Autodesk Fusion 360 part; units mm, degrees
(part 2 of 2)
sketch "Sketch1 (6)" plane through (0, 0, 0) normal (0, 1, 0) x (1, 0, 0) in component "Peça P3"
  line L0 (-20, -6) -> (-20, 10)
  line L1 (36, 30) -> (-36, 30)
  line L2 (-20, 10) -> (20, 10)
  line L3 (40, -6) -> (40, 26)
  arc A0 (-40, -6) -> (-36, -10) centre (-36, -6) ccw
  arc A1 (20, -6) -> (24, -10) centre (24, -6) ccw
  arc A2 (-24, -10) -> (-20, -6) centre (-24, -6) ccw
  line L4 (-40, 26) -> (-40, -6)
  line L5 (20, 10) -> (20, -6)
  arc A3 (-36, 30) -> (-40, 26) centre (-36, 26) ccw
  arc A4 (40, 26) -> (36, 30) centre (36, 26) ccw
  line L6 (24, -10) -> (36, -10)
  arc A5 (36, -10) -> (40, -6) centre (36, -6) ccw
  line L7 (-36, -10) -> (-24, -10)
  point P0 (-20, -10)
  point P1 (40, -10)
  point P2 (-40, -10)
  point P3 (-40, 30)
  dimension "d21" = 80
  dimension "d22" = 40
  dimension "d23" = 40
  dimension "d24" = 20
  dimension "d25" = 4
  dimension "d26" = 4
  dimension "d27" = 4
  dimension "d28" = 4
  dimension "d29" = 4
  dimension "d30" = 4
  constraint horizontal L1
  constraint perpendicular L1 L4
  constraint parallel L1 L7
  constraint parallel L3 L4
  constraint parallel L0 L5
  constraint coincident P3 L1
  constraint coincident P3 L4
  constraint tangent L1 A3
  constraint tangent L4 A3
  constraint tangent L1 A4
  constraint tangent L3 A4
  constraint collinear L6 L7
  constraint coincident P0 L0
  constraint coincident P0 L7
  constraint tangent L0 A2
  constraint tangent A2 L7
  constraint tangent A1 L5
  constraint tangent A1 L6
  constraint coincident P1 L3
  constraint coincident P1 L6
  constraint tangent L3 A5
  constraint tangent L6 A5
  constraint coincident P2 L4
  constraint coincident P2 L7
  constraint tangent A0 L4
  constraint tangent A0 L7
  measures "d21" distance of P1 P2
  measures "d22" distance of P2 P3
  measures "d23" distance of L2.end L0.end
  measures "d24" distance of P0 L0.end
  measures "d25" radius of A3
  measures "d26" radius of A4
  measures "d27" radius of A2
  measures "d28" radius of A1
  measures "d29" radius of A5
  measures "d30" radius of A0
extrude "Extrude2" add sketch "Sketch1" along normal blind 15 makes body 1 in component "Peça P1"
extrude "Extrude2'" add sketch "Sketch1 (2)" along normal blind 15 separate body makes body 2 in component "Peça P2"
extrude "Extrude2''" add sketch "Sketch1 (3)" along normal blind 15 separate body makes body 3 in component "Peça P3"
extrude "Extrude2'''" add sketch "Sketch1 (4)" along normal blind 15 separate body makes body 4 in component "Peça P4"
extrude "Extrude2''''" add sketch "Sketch1 (5)" along normal blind 15 separate body makes body 5 in component "Peça G1"
extrude "Extrude1" add sketch "Sketch G2" along normal blind 15 separate body makes body 6 in component "Peça G2"
extrude "Extrude1'" add sketch "Sketch G3" along normal blind 15 separate body makes body 7 in component "Peça G3"
extrude "Extrude1''" add sketch "Sketch G4" along normal blind 15 separate body makes body 8 in component "Peça G4"
sketch "Sketch C1" plane through (0, 0, 0) normal (0, 1, 0) x (1, 0, 0) in component "Peça C1"
  line L0 (-40.0297, 4.2229) -> (-40.0318, 36.0014)
  line L1 (-36.0335, 40.0017) -> (-4.255, 40.0151)
  arc A0 (-0.2817, 44.4612) -> (-44.4739, 0.2474) centre (-40.0321, 40) ccw
  arc A1 (-4.255, 40.0151) -> (-0.2817, 44.4612) centre (-4.2567, 44.0151) ccw
  arc A2 (-36.0335, 40.0017) -> (-40.0318, 36.0014) centre (-36.0318, 36.0017) ccw
  arc A3 (-44.4739, 0.2474) -> (-40.0297, 4.2229) centre (-44.0297, 4.2226) ccw
  line L2 (-65, 60) -> (-65, 25)
  line L3 (-70, 25) -> (-70, 60)
  line L4 (-45, 70) -> (-45, 45)
  line L5 (-50, 45) -> (-50, 70)
  line L6 (-30, 75) -> (-30, 45)
  line L7 (-35, 45) -> (-35, 75)
  line L8 (-55, 65) -> (-55, 35)
  line L9 (-60, 35) -> (-60, 65)
  arc A4 (-30, 75) -> (-35, 75) centre (-32.5, 75) ccw
  arc A5 (-35, 45) -> (-30, 45) centre (-32.5, 45) ccw
  arc A6 (-50, 45) -> (-45, 45) centre (-47.5, 45) ccw
  arc A7 (-45, 70) -> (-50, 70) centre (-47.5, 70) ccw
  arc A8 (-55, 65) -> (-60, 65) centre (-57.5, 65) ccw
  arc A9 (-60, 35) -> (-55, 35) centre (-57.5, 35) ccw
  arc A10 (-70, 25) -> (-65, 25) centre (-67.5, 25) ccw
  arc A11 (-65, 60) -> (-70, 60) centre (-67.5, 60) ccw
  point P0 (-40.0294, 0)
  point P1 (-40.0321, 40)
  point P2 (0, 20)
  dimension "d415" = 40
  dimension "d416" = 4
  dimension "d417" = 4
  dimension "d418" = 4
  dimension "d419" = 2.5
  dimension "d420" = 4.2567
  dimension "d421" = 15.9849
  dimension "d422" = 9.0151
  dimension "d423" = 0.9849
  dimension "d424" = 63.2433
  dimension "d425" = 53.2433
  dimension "d426" = 43.2433
  dimension "d427" = 28.2433
  dimension "d428" = 89.976
  dimension "d429" = 30
  dimension "d430" = 25
  dimension "d431" = 24.0151
  dimension "d432" = 39.7924
  dimension "d433" = 35
  constraint coincident P1 A0.centre
  constraint tangent A0 A1
  constraint tangent L1 A1
  constraint coincident P1 L0
  constraint coincident P1 L1
  constraint tangent L0 A2
  constraint tangent L1 A2
  constraint coincident P0 L0
  constraint coincident P0 A0
  constraint tangent L0 A3
  constraint tangent A0 A3
  constraint vertical L2
  constraint vertical L3
  constraint vertical L4
  constraint vertical L5
  constraint vertical L6
  constraint vertical L7
  constraint vertical L8
  constraint vertical L9
  constraint tangent L3 A11
  constraint tangent L3 A10
  constraint tangent L9 A8
  constraint tangent L9 A9
  constraint tangent L4 A7
  constraint tangent L5 A6
  constraint tangent L7 A4
  constraint tangent L6 A5
  constraint tangent L2 A10
  constraint tangent L2 A11
  constraint tangent L8 A9
  constraint tangent L8 A8
  constraint tangent L5 A7
  constraint tangent L4 A6
  constraint tangent L7 A5
  constraint tangent L6 A4
  constraint horizontal L5.start L7.start
  constraint equal A4 A6
  constraint equal A4 A8
  constraint equal A4 A10
  constraint equal L6 L8
  constraint vertical origin P2
  constraint horizontal origin P0
  measures "d415" distance of P0 A0.centre
  measures "d416" radius of A1
  measures "d417" radius of A2
  measures "d418" radius of A3
  measures "d419" radius of A5
  measures "d420" horizontal distance of origin A1.centre
  measures "d421" vertical distance of A1.centre A11.centre
  measures "d422" vertical distance of A1.centre A9.centre
  measures "d423" vertical distance of A1.centre A5.centre
  measures "d424" horizontal distance of A1.centre A11.centre
  measures "d425" horizontal distance of A1.centre A9.centre
  measures "d426" horizontal distance of A1.centre A6.centre
  measures "d427" horizontal distance of A1.centre A5.centre
  measures "d428" angle of L1 L3
  measures "d429" vertical distance of A4.centre A5.centre
  measures "d430" vertical distance of A7.centre A6.centre
  measures "d431" vertical distance of P2 A1.centre
  measures "d432" vertical distance of A1.centre A3.centre
  measures "d433" vertical distance of A11.centre A10.centre
sketch "Sketch C2" plane through (0, 0, 0) normal (0, 1, 0) x (1, 0, 0) in component "Peça C2"
  arc A0 (-44.4661, 0.2446) -> (-40.0232, 4.2216) centre (-44.0232, 4.22) ccw
  line L0 (-40.0232, 4.2216) -> (-40.0355, 35.9987)
  line L1 (-36.037, 40.0002) -> (-4.2599, 40.0124)
  arc A1 (-4.2599, 40.0124) -> (-0.2864, 44.4584) centre (-4.2615, 44.0124) ccw
  arc A2 (-0.2864, 44.4584) -> (-44.4661, 0.2446) centre (-40.037, 39.9987) ccw
  arc A3 (-36.037, 40.0002) -> (-40.0355, 35.9987) centre (-36.0355, 36.0002) ccw
  circle A4 centre (-59.1399, 63.4514) radius 5
  circle A5 centre (-45.0248, 68.2909) radius 5
  circle A6 centre (-66.8025, 53.3691) radius 3
  circle A7 centre (-47.0412, 53.7724) radius 3
  circle A8 centre (-49.0577, 13.0401) radius 5
  circle A9 centre (-61.7613, 37.2375) radius 5
  circle A10 centre (-33.7327, 60.6284) radius 3
  circle A11 centre (-13.1649, 50.3445) radius 6
  circle A12 centre (-52.8889, 45.9083) radius 4
  circle A13 centre (-27.0784, 67.2827) radius 4
  circle A14 centre (-29.2965, 49.9412) radius 4
  circle A15 centre (-73.0535, 43.8918) radius 3
  circle A16 centre (-49.8643, 28.5668) radius 5
  circle A17 centre (-64.3827, 23.929) radius 4
  circle A18 centre (-71.4403, 32.5997) radius 4
  point P0 (-40.037, 39.9987)
  point P1 (-40.0216, -0.0013)
  point P2 (-0.0047, 19.9974)
  point P3 (-0.0047, -0.0013)
  dimension "d434" = 40
  dimension "d435" = 4
  dimension "d436" = 4
  dimension "d437" = 4
  dimension "d439" = 4.2567
  dimension "d450" = 24.0151
  dimension "d451" = 39.7924
  dimension "d453" = 10
  dimension "d454" = 10
  dimension "d455" = 6
  dimension "d456" = 6
  dimension "d457" = 10
  dimension "d458" = 10
  dimension "d459" = 6
  dimension "d460" = 12
  dimension "d461" = 8
  dimension "d462" = 8
  dimension "d463" = 8
  dimension "d464" = 6
  dimension "d465" = 10
  dimension "d466" = 8
  dimension "d467" = 8
  dimension "d468" = 4.2615
  dimension "d469" = 67.1788
  dimension "d470" = 62.541
  dimension "d471" = 60.1213
  dimension "d472" = 57.4999
  dimension "d473" = 54.8785
  dimension "d474" = 48.6275
  dimension "d475" = 45.6028
  dimension "d476" = 44.7962
  dimension "d477" = 42.7798
  dimension "d478" = 40.7633
  dimension "d479" = 29.4712
  dimension "d480" = 25.035
  dimension "d481" = 22.8169
  dimension "d482" = 8.9034
  dimension "d483" = 90
  dimension "d484" = 44.0124
  dimension "d485" = 68.792
  dimension "d486" = 30.9723
  dimension "d487" = 24.2784
  dimension "d488" = 23.2702
  dimension "d489" = 20.0835
  dimension "d490" = 19.439
  dimension "d491" = 16.6159
  dimension "d492" = 15.4457
  dimension "d493" = 11.4128
  dimension "d494" = 9.76
  dimension "d495" = 9.3567
  dimension "d496" = 6.7749
  dimension "d497" = 6.332
  dimension "d498" = 5.9287
  dimension "d499" = 1.8958
  dimension "d500" = 0.1206
  constraint coincident P0 A2.centre
  constraint tangent A1 A2
  constraint tangent L1 A1
  constraint coincident P0 L0
  constraint coincident P0 L1
  constraint tangent L0 A3
  constraint tangent L1 A3
  constraint coincident P1 L0
  constraint coincident P1 A2
  constraint tangent A0 L0
  constraint tangent A0 A2
  constraint vertical P2 P3
  constraint horizontal P1 P3
  measures "d434" distance of P0 P1
  measures "d435" radius of A1
  measures "d436" radius of A3
  measures "d437" radius of A0
  measures "d439" horizontal distance of A1.centre P3
  measures "d450" vertical distance of P2 A1.centre
  measures "d451" vertical distance of A1.centre A0.centre
  measures "d453" diameter of A4
  measures "d454" diameter of A5
  measures "d455" diameter of A6
  measures "d456" diameter of A7
  measures "d457" diameter of A8
  measures "d458" diameter of A9
  measures "d459" diameter of A10
  measures "d460" diameter of A11
  measures "d461" diameter of A12
  measures "d462" diameter of A13
  measures "d463" diameter of A14
  measures "d464" diameter of A15
  measures "d465" diameter of A16
  measures "d466" diameter of A17
  measures "d467" diameter of A18
  measures "d468" horizontal distance of origin A1.centre
  measures "d469" horizontal distance of A1.centre A18.centre
  measures "d470" horizontal distance of A1.centre A6.centre
  measures "d471" horizontal distance of A1.centre A17.centre
  measures "d472" horizontal distance of A1.centre A9.centre
  measures "d473" horizontal distance of A1.centre A4.centre
  measures "d474" horizontal distance of A1.centre A12.centre
  measures "d475" horizontal distance of A1.centre A16.centre
  measures "d476" horizontal distance of A1.centre A8.centre
  measures "d477" horizontal distance of A1.centre A7.centre
  measures "d478" horizontal distance of A1.centre A5.centre
  measures "d479" horizontal distance of A1.centre A10.centre
  measures "d480" horizontal distance of A1.centre A14.centre
  measures "d481" horizontal distance of A1.centre A13.centre
  measures "d482" horizontal distance of A1.centre A11.centre
  measures "d483" angle of L0 L1
  measures "d484" vertical distance of origin A1.centre
  measures "d485" horizontal distance of A1.centre A15.centre
  measures "d486" vertical distance of A1.centre A8.centre
  measures "d487" vertical distance of A1.centre A5.centre
  measures "d488" vertical distance of A1.centre A13.centre
  measures "d489" vertical distance of A1.centre A17.centre
  measures "d490" vertical distance of A1.centre A4.centre
  measures "d491" vertical distance of A1.centre A10.centre
  measures "d492" vertical distance of A1.centre A16.centre
  measures "d493" vertical distance of A1.centre A18.centre
  measures "d494" vertical distance of A1.centre A7.centre
  measures "d495" vertical distance of A1.centre A6.centre
  measures "d496" vertical distance of A1.centre A9.centre
  measures "d497" vertical distance of A1.centre A11.centre
  measures "d498" vertical distance of A1.centre A14.centre
  measures "d499" vertical distance of A1.centre A12.centre
  measures "d500" vertical distance of A1.centre A15.centre
sketch "Sketch C3" plane through (0, 0, 0) normal (0, 1, 0) x (1, 0, 0) in component "Peça C3"
  arc A0 (-4.2599, 40.0124) -> (-0.2864, 44.4584) centre (-4.2615, 44.0124) ccw
  arc A1 (-0.2864, 44.4584) -> (-44.4661, 0.2446) centre (-40.037, 39.9987) ccw
  line L0 (-36.037, 40.0002) -> (-4.2599, 40.0124)
  arc A2 (-36.037, 40.0002) -> (-40.0355, 35.9987) centre (-36.0355, 36.0002) ccw
  arc A3 (-44.4661, 0.2446) -> (-40.0232, 4.2216) centre (-44.0232, 4.22) ccw
  line L1 (-40.0232, 4.2216) -> (-40.0355, 35.9987)
  arc A4 (-4.8251, 44.5122) -> (-44.5234, 4.7833) centre (-40.037, 39.9987) ccw
  line L2 (-44.5234, 4.7833) -> (-44.5355, 35.9969)
  arc A5 (-36.0387, 44.5002) -> (-44.5355, 35.9969) centre (-36.0355, 36.0002) ccw
  line L3 (-36.0387, 44.5002) -> (-4.8251, 44.5122)
  point P0 (-40.0216, -0.0013)
  point P1 (-0.0047, 19.9974)
  point P2 (-40.037, 39.9987)
  point P3 (-0.0047, -0.0013)
  dimension "d501" = 40
  dimension "d502" = 4
  dimension "d503" = 4
  dimension "d504" = 4
  dimension "d505" = 4.2567
  dimension "d506" = 24.0151
  dimension "d507" = 39.7924
  dimension "d523" = 4.2615
  dimension "d538" = 90
  dimension "d539" = 44.0124
  dimension "d556" = -4.5
  constraint coincident P2 A1.centre
  constraint tangent A0 A1
  constraint tangent A0 L0
  constraint coincident P2 L1
  constraint coincident P2 L0
  constraint tangent A2 L1
  constraint tangent L0 A2
  constraint coincident P0 L1
  constraint coincident P0 A1
  constraint tangent A3 L1
  constraint tangent A1 A3
  constraint vertical P1 P3
  constraint horizontal P0 P3
  measures "d501" distance of P0 P2
  measures "d502" radius of A0
  measures "d503" radius of A2
  measures "d504" radius of A3
  measures "d505" horizontal distance of P3 A0.centre
  measures "d506" vertical distance of P1 A0.centre
  measures "d507" vertical distance of A3.centre A0.centre
  measures "d523" horizontal distance of origin A0.centre
  measures "d538" angle of L0 L1
  measures "d539" vertical distance of origin A0.centre
extrude "Extrude1'''" add sketch "Sketch C1" along normal blind 15 separate body makes body 9 in component "Peça C1"
extrude "Extrude1''''" add sketch "Sketch C2" along normal blind 15 separate body makes body 10 in component "Peça C2"
extrude "Extrude1'''''" add sketch "Sketch C3" along normal blind 15 separate body makes body 11 in component "Peça C3"
other "Arrange1"
move_body "Move1" bodies 3 to x (-1, 0, 0) y (0, 1, 0) z (0, 0, -1) at (-80, 0, -60) in component "Peça P3"
move_body "Move1'" bodies 4 to x (0, 0, -1) y (0, 1, 0) z (1, 0, 0) at (-10, 0, -70) in component "Peça P4"
move_body "Move2" bodies 4 to x (0, 0, -1) y (0, 1, 0) z (1, 0, 0) at (70, 0, -150) in component "Peça P4"
move_body "Move3" bodies 4 to x (1, 0, 0) y (0, 1, 0) z (0, 0, 1) at (0, 0, 250) in component "Peça P4"
move_body "Move1''" bodies 5 to x (-1, 0, 0) y (0, 1, 0) z (0, 0, -1) at (-221, 0, -80) in component "Peça G1"
move_body "Move2'" bodies 3 to x (0, 1, 0) y (-1, 0, 0) z (0, 0, 1) at (-140, 140, 0) in component "Peça P3"
move_body "Move1'''" bodies 2 to x (0, 1, 0) y (-1, 0, 0) z (0, 0, 1) at (-101.7071, 101.7071, 0) in component "Peça P2"
move_body "Move4" bodies 4 to x (0, 1, 0) y (-1, 0, 0) z (0, 0, 1) at (-101.7071, 101.7071, 0) in component "Peça P4"
move_body "Move2''" bodies 5 to x (0, 1, 0) y (-1, 0, 0) z (0, 0, 1) at (-230.5, 230.5, 0) in component "Peça G1"
move_body "Move2'''" bodies 2 to x (1, 0, 0) y (0, 1, 0) z (0, 0, 1) at (0, -2, 0) in component "Peça P2"
move_body "Move5" bodies 4 to x (1, 0, 0) y (0, 1, 0) z (0, 0, 1) at (0, -1, 0) in component "Peça P4"
move_body "Move3'" bodies 2 to x (1, 0, 0) y (0, 1, 0) z (0, 0, 1) at (0, 0.5, 0) in component "Peça P2"
move_body "Move6" bodies 4 to x (1, 0, 0) y (0, 1, 0) z (0, 0, 1) at (0, -0.5, 0) in component "Peça P4"
move_body "Move3''" bodies 3 to x (1, 0, 0) y (0, 1, 0) z (0, 0, 1) at (0, -60, -100) in component "Peça P3"
move_body "Move4'" bodies 2 to x (1, 0, 0) y (0, 1, 0) z (0, 0, 1) at (0, -60, -100) in component "Peça P2"
move_body "Move7" bodies 4 to x (1, 0, 0) y (0, 1, 0) z (0, 0, 1) at (0, 60, 100) in component "Peça P4"
move_body "Move3'''" bodies 5 to x (1, 0, 0) y (0, 1, 0) z (0, 0, 1) at (0, -60, -100) in component "Peça G1"
move_body "Move1''''" bodies 9 to x (1, 0, 0) y (0, 1, 0) z (0, 0, 1) at (150, 0, 0) in component "Peça C1"
move_body "Move2''''" bodies 9 to x (-1, 0, 0) y (0, 1, 0) z (0, 0, -1) at (139.9358, 0, 10) in component "Peça C1"
move_body "Move1'''''" bodies 6 to x (1, 0, 0) y (0, 1, 0) z (0, 0, 1) at (0, 0, 150) in component "Peça G2"
move_body "Move2'''''" bodies 6 to x (0, 0, 1) y (0, 1, 0) z (-1, 0, 0) at (-0.5, 0, 220.5) in component "Peça G2"
move_body "Move3''''" bodies 6 to x (1, 0, 0) y (0, 1, 0) z (0, 0, 1) at (40, 0, -50) in component "Peça G2"
move_body "Move4''" bodies 6 to x (1, 0, 0) y (0, 1, 0) z (0, 0, 1) at (0, 0, -10) in component "Peça G2"
move_body "Move1''''''" bodies 1 to x (1, 0, 0) y (0, 1, 0) z (0, 0, 1) at (0, 90, 0) in component "Peça P1"
move_body "Move2''''''" bodies 1 to x (1, 0, 0) y (0, 1, 0) z (0, 0, 1) at (-180, 0, 0) in component "Peça P1"
move_body "Move3'''''" bodies 1 to x (1, 0, 0) y (0, 0, -1) z (0, 1, 0) at (280, 120, 60) in component "Peça P1"
move_body "Move4'''" bodies 1 to x (1, 0, 0) y (0, 1, 0) z (0, 0, 1) at (10, 0, 0) in component "Peça P1"
move_body "Move1'''''''" bodies 7 to x (1, 0, 0) y (0, 0, 1) z (0, -1, 0) at (-50, -40, -40) in component "Peça G3"
move_body "Move2'''''''" bodies 7 to x (1, 0, 0) y (0, 1, 0) z (0, 0, 1) at (-1, 0, 0) in component "Peça G3"
move_body "Move1''''''''" bodies 8 to x (1, 0, 0) y (0, 1, 0) z (0, 0, 1) at (0, 0, 210) in component "Peça G4"
move_body "Move2''''''''" bodies 8 to x (0, 1, 0) y (-1, 0, 0) z (0, 0, 1) at (-110.5, 110.5, 0) in component "Peça G4"
move_body "Move3''''''" bodies 8 to x (-1, 0, 0) y (0, 1, 0) z (0, 0, -1) at (-251, 0, 340) in component "Peça G4"
move_body "Move4''''" bodies 8 to x (1, 0, 0) y (0, 1, 0) z (0, 0, 1) at (0, 0, 50) in component "Peça G4"
move_body "Move5'" bodies 8 to x (1, 0, 0) y (0, 1, 0) z (0, 0, 1) at (0, 0, -30) in component "Peça G4"
move_body "Move1'''''''''" bodies 10 to x (0, 0, 1) y (0, 1, 0) z (-1, 0, 0) at (-50.0357, 0, 0.0383) in component "Peça C2"
move_body "Move2'''''''''" bodies 10 to x (1, 0, 0) y (0, 1, 0) z (0, 0, 1) at (0, 0, 11.5) in component "Peça C2"
move_body "Move1''''''''''" bodies 11 to x (0, 1, 0) y (-1, 0, 0) z (0, 0, 1) at (-80.037, 80.037, 0) in component "Peça C3"
move_body "Move2''''''''''" bodies 11 to x (1, 0, 0) y (0, 0, 1) z (0, -1, 0) at (0, -79.9987, -79.9987) in component "Peça C3"
move_body "Move3'''''''" bodies 11 to x (1, 0, 0) y (0, 1, 0) z (0, 0, 1) at (0, 100, 150) in component "Peça C3"
move_body "Move3''''''''" bodies 10 to x (1, -0.000385, -0.000385) y (0.000385, 0, 1) z (-0.000385, -1, 0) at (0.0366, 125.0031, 95.0031) in component "Peça C2"
move_body "Move4'''''" bodies 11 to x (0, 0, -1) y (0, 1, 0) z (1, 0, 0) at (-165.0383, 0, -25.0357) in component "Peça C3"
move_body "Move4''''''" bodies 3 to x (0, 0, -1) y (0, 1, 0) z (1, 0, 0) at (-104.0059, 0, -205.9941) in component "Peça P3"
move_body "Move5''" bodies 1 to x (0, 0.000067, -1) y (-0.000067, 1, 0.000067) z (1, 0.000067, 0) at (140.0056, -0.0054, 79.9935) in component "Peça P1"
move_body "Move5'''" bodies 2 to x (0, 0, -1) y (0, 1, 0) z (1, 0, 0) at (-125.0059, 0, -108.4083) in component "Peça P2"
move_body "Move8" bodies 4 to x (0, 0, 1) y (0, 1, 0) z (-1, 0, 0) at (-15.0059, 0, 218.4083) in component "Peça P4"
move_body "Move6'" bodies 8 to x (0, 0, -1) y (0, 1, 0) z (1, 0, 0) at (-250.4996, 0, -30.5005) in component "Peça G4"
move_body "Move5''''" bodies 6 to x (1, 0, 0) y (0, 0, 1) z (0, -1, 0) at (0, 125.0069, 95.0069) in component "Peça G2"
move_body "Move3'''''''''" bodies 7 to x (0, -0.000067, -1) y (0.000067, 1, -0.000067) z (1, -0.000067, 0) at (-61.4956, -0.0095, -141.5035) in component "Peça G3"
move_body "Move3''''''''''" bodies 9 to x (1, 0, 0) y (0, 0, 1) z (0, -1, 0) at (0, 125.0069, 95.0069) in component "Peça C1"
move_body "Move4'''''''" bodies 5 to x (0, 0, -1) y (0, 1, 0) z (1, 0, 0) at (-165.5059, 0, -325.4941) in component "Peça G1"
extrude "Extrude1''''''" add 1 faces at (-95.5, -32.4931, 100.0069) faces seen with x (0, 1, 0.000067) y (-1, 0, 0) z (0, -0.000067, 1) at (-95.5, 110.5038, 0) along direction (1, 0, 0) blind 275 separate body on bodies 6 makes body 12 in component "Light for render"
move_body "Move1'''''''''''" bodies 12 to x (1, 0, 0) y (0, 1, 0) z (0, 0, 1) at (0, 175, 250) in component "Light for render"
extrude "Extrude2'''''" add 1 faces at (120.3264, 209.9971, 350.0019) along direction (0, 1, 0.000067) blind 275 on bodies 12 bodies 12 in component "Light for render"
move_body "Move2'''''''''''" bodies 12 to x (0.707107, 0, 0.707107) y (0, 1, 0) z (-0.707107, 0, 0.707107) at (-274.5025, 0, 145.6008) in component "Light for render"
move_body "Move3'''''''''''" bodies 12 to x (1, 0, 0) y (0, 1, 0) z (0, 0, 1) at (0, 0, 100) in component "Light for render"
move_body "Move4''''''''" bodies 12 to x (0.906308, -0.422618, 0) y (0.422618, 0.906308, 0) z (0, 0, 1) at (-129.8142, -225.5614, 0) in component "Light for render"
move_body "Move5'''''" bodies 12 to x (1, 0, 0) y (0, 0.906308, -0.422618) z (0, 0.422618, 0.906308) at (0, -29.3209, 81.1354) in component "Light for render"
move_body "Move6''" bodies 12 to x (1, 0, 0) y (0, 1, 0) z (0, 0, 1) at (0, 0, 300) in component "Light for render"
move_body "Move7'" bodies 12 to x (1, 0, 0) y (0, 1, 0) z (0, 0, 1) at (0, 0, 300) in component "Light for render"
move_body "Move8'" bodies 12 to x (-0.173648, 0, -0.984808) y (-0.336824, 0.939693, 0.059391) z (0.925417, 0.34202, -0.163176) at (-792.9971, -286.4144, 455.4732) in component "Light for render"
component "Peça P2" placed x (1, 0, 0) y (0, 1, 0.000067) z (0, -0.000067, 1) at (6.2071, 80.2041, 101.7061)
component "Peça P3" placed x (1, 0, 0) y (0, 1, 0.000067) z (0, -0.000067, 1) at (44.5, 80.2001, 160.999)
component "Peça P4" placed x (1, 0, 0) y (0, -1, -0.000067) z (0, 0.000067, -1) at (6.2071, 200.1967, 211.7141)
component "Peça G1" placed x (1, 0, 0) y (0, 1, 0.000067) z (0, -0.000067, 1) at (135, 80.1982, 189.999)
component "Peça G2" placed x (0, 1, 0.000067) y (-1, 0, 0) z (0, -0.000067, 1) at (-95.5, 110.5038, 0)
component "Peça G3" placed x (0, 0.000067, -1) y (0.000067, 1, 0.000067) z (1, -0.000067, 0) at (-70.4961, 99.0005, 8.5066)
component "Peça G4" placed x (1, 0, 0) y (0, 1, 0.000067) z (0, -0.000067, 1) at (30, 40.0038, 0.0027)
component "Peça C1" placed x (0, 1, 0.000067) y (-1, 0, 0) z (0, -0.000067, 1) at (-95.5, 110.2426, 0)
component "Peça C2" placed x (0, 1, 0.000452) y (-1, 0, 0) z (0, -0.000452, 1) at (-95.5, 170.4396, 0.0078)
component "Peça C3" placed x (1, 0, 0) y (0, 1, 0.000067) z (0, -0.000067, 1) at (-15.463, 100.0006, 40.0049)
component "Peça P1" placed x (0, -0.000067, 1) y (0.000067, 1, 0.000067) z (-1, 0.000067, 0) at (-140.506, -49.9942, -0.0033)
component "Arrange1" placed x (1, 0, 0) y (0, 1, 0) z (0, 0, 1) at (0, 0, 0)
component "Light for render" placed x (1, 0, 0) y (0, 1, 0) z (0, 0, 1) at (0, 0, 0)
component "Peças - Texturitas Renders v6" placed x (1, 0, 0) y (0, 1, 0) z (0, 0, 1) at (0, 0, 0) in component "Peça G4"
component "Envelope1(Qty: 1)" placed x (0, 0, 1) y (1, 0, 0) z (0, 1, 0) at (0, 0, 0) in component "Arrange1"
component "Peça P1" placed x (0, -1, 0) y (0, 0, 1) z (-1, 0, 0) at (89.5145, 264.847, -90) in component "Envelope1(Qty: 1)"
component "Peça P2" placed x (0, 1, 0) y (0, 0, 1) z (1, 0, 0) at (82.7, 245.3325, 0) in component "Envelope1(Qty: 1)"
component "Peça P3" placed x (0, 1, 0) y (0, 0, 1) z (1, 0, 0) at (82.7, 418.0325, 0) in component "Envelope1(Qty: 1)"
component "Peça P4" placed x (0, 1, 0) y (0, 0, 1) z (1, 0, 0) at (82.7, 331.6825, 0) in component "Envelope1(Qty: 1)"
component "Peça G1" placed x (0, 0, 1) y (0, 1, 0) z (-1, 0, 0) at (-133.65, 445.4, 245.5) in component "Envelope1(Qty: 1)"
component "Peça G2" placed x (-1, 0, 0) y (0, 0, 1) z (0, 1, 0) at (-64.15, -43.65, 0) in component "Envelope1(Qty: 1)"
component "Peça G3" placed x (0, 1, 0) y (0, 0, 1) z (1, 0, 0) at (46.35, 243.2, 0) in component "Envelope1(Qty: 1)"
component "Peça G4" placed x (0, 1, 0) y (0, 0, 1) z (1, 0, 0) at (46.35, 369.55, 0) in component "Envelope1(Qty: 1)"
component "Peça C1" placed x (0, 1, 0) y (0, 0, 1) z (1, 0, 0) at (23.028, 128.7624, 0) in component "Envelope1(Qty: 1)"
component "Peça C2" placed x (0, -1, 0) y (0, 0, 1) z (-1, 0, 0) at (12.6858, 505.7711, 0) in component "Envelope1(Qty: 1)"
component "Peça C3" placed x (0, -1, 0) y (0, 0, 1) z (-1, 0, 0) at (32.8757, 6.263, 0) in component "Envelope1(Qty: 1)"
equation "opcional_Esp = 15 mm"
equation "esp = 16 mm"
named bodies: "Body C2"
